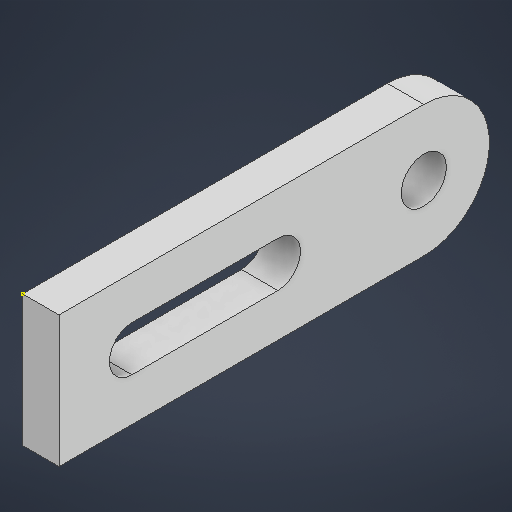
# Autodesk Inventor part: roller bracket
Saved by Autodesk Inventor 2027 (Build 310192000, 192)
## iProperties
Created: 2026-07-15
Part Number: roller bracket
Material: Generic
Document SubType Name: Modeling
Designer: ratik
Density: 1 g/cm^3
Appearance: Default
Author: ratik
Autodesk Inventor part; units mm, degrees
ref_plane "YZ Plane" through (0, 0, 0) normal (1, 0, 0) x (0, 1, 0)
ref_plane "XZ Plane" through (0, 0, 0) normal (0, 1, 0) x (-1, 0, 0)
ref_plane "XY Plane" through (0, 0, 0) normal (0, 0, 1) x (1, 0, 0)
sketch "Sketch1" plane through (0, 0, 0) normal (1, 0, 0) x (0, 1, 0)
  point P0 (0, 0)
sketch "Sketch2" plane through (0, 0, 0) normal (1, 0, 0) x (0, 1, 0)
  line L0 (0, 0) -> (-18, 0)
  line L1 (-18, 0) -> (-18, -50)
  line L2 (0, -50) -> (0, 0)
  arc A0 (-18, -50) -> (0, -50) centre (-9, -50) ccw
  point P0 (-4.8185, -57.9696)
  dimension "d0" = 18
  dimension "d1" = 50
  dimension "d4" = 18
  constraints: 6 end point, 3 point on circle, 1 centre point, 1 horizontal, 1 parallel, 1 perpendicular
  measures "d0" distance between parallel lines of L2 L1
  measures "d1" distance of L0.end L1.end
  measures "d4" diameter of A0
extrude "Extrusion1" add sketch "Sketch2" along normal blind 5
sketch "Sketch3" plane through (5, 0, 0) normal (1, 0, 0) x (0, 0, -1)
  arc A0 (50, -18) -> (50, 0) centre (50, -9) ccw projected
  circle A1 centre (50, -9) radius 3.1
  arc A2 (10, -5.9) -> (10, -12.1) centre (10, -9) ccw
  arc A3 (30, -12.1) -> (30, -5.9) centre (30, -9) ccw
  line L0 (10, -5.9) -> (30, -5.9)
  line L1 (10, -12.1) -> (30, -12.1)
  line L2 (0, 0) -> (0, -18) projected
  dimension "d5" = 6.2
  dimension "d6" = 6.2
  dimension "d7" = 6.2
  dimension "d8" = 10
  dimension "d9" = 20
  constraints: 4 end point, 4 point on circle, 3 centre point, 2 tangent, 1 coincident, 1 horizontal, 1 parallel
  measures "d5" diameter of A1
  measures "d6" diameter of A2
  measures "d7" diameter of A3
  measures "d8" distance from line of L2 A2.centre
  measures "d9" distance of A2.centre A3.centre
extrude "Extrusion2" cut sketch "Sketch3" against normal through all
body "Solid1"
